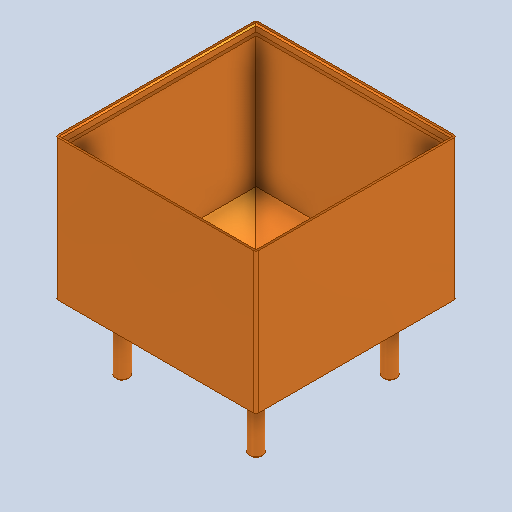
# Autodesk Inventor part: coffe container
Saved by Autodesk Inventor 2023 (Build 270158000, 158)
## iProperties
Created: 2022-11-26
Part Number: coffe container
Material: Gold
Document SubType Name: Modeling
Designer: abdul
Density: 19.3 g/cm^3
Appearance: Metal 1600F Hot
Author: abdul
Autodesk Inventor part; units mm, degrees
ref_plane "YZ Plane" through (0, 0, 0) normal (1, 0, 0) x (0, 1, 0)
ref_plane "XZ Plane" through (0, 0, 0) normal (0, 1, 0) x (-1, 0, 0)
ref_plane "XY Plane" through (0, 0, 0) normal (0, 0, 1) x (1, 0, 0)
sketch "Sketch1" plane through (0, 0, 0) normal (0, 1, 0) x (-1, 0, 0)
  line L0 (75, 75) -> (-75, 75)
  line L1 (-75, 75) -> (-75, -75)
  line L2 (-75, -75) -> (75, -75)
  line L3 (75, -75) -> (75, 75)
  point P0 (0, 0)
  dimension "d0" = 150
  dimension "d1" = 150
  dimension "d6" = 75
  dimension "d7" = 75
  constraints: 8 end point, 2 parallel, 1 horizontal, 1 perpendicular
  measures "d0" distance of L2.end L1.end
  measures "d1" distance of L1.end L0.end
  measures "d6" distance from line of L0 point (0, 0)
  measures "d7" distance from line of L3 point (0, 0)
extrude "Extrusion1" add sketch "Sketch1" along normal blind 100
sketch "Sketch2" plane through (0, 100, 0) normal (0, 1, 0) x (1, 0, 0)
  line L0 (-70, -70) -> (70, -70)
  line L1 (70, -70) -> (70, 70)
  line L2 (70, 70) -> (-70, 70)
  line L3 (-70, 70) -> (-70, -70)
  line L4 (75, 75) -> (-75, 75) projected
  line L5 (-75, -75) -> (75, -75) projected
  line L6 (-75, 75) -> (-75, -75) projected
  line L7 (75, -75) -> (75, 75) projected
  point P0 (0, 0)
  dimension "d8" = 140
  dimension "d9" = 140
  dimension "d10" = 5
  dimension "d11" = 5
  constraints: 8 end point, 6 parallel, 1 horizontal, 1 perpendicular
  measures "d8" distance of L2.end L1.end
  measures "d9" distance of L1.end L0.end
  measures "d10" distance between parallel lines of L5 L0
  measures "d11" distance between parallel lines of L6 L3
extrude "Extrusion2" cut sketch "Sketch2" against normal blind 90 contours L3 L2 L1 L0
ref_plane "Work Plane1" through (0, -50, 0) normal (0, -1, 0) x (1, 0, 0)
sketch "Sketch3" plane through (0, -50, 0) normal (0, -1, 0) x (1, 0, 0)
  circle A0 centre (0, 0) radius 15
  dimension "d15" = 30
  constraints: 1 centre point, 1 coincident
  measures "d15" diameter of A0
loft "Loft1" add profiles "Sketch3" section 2 edges at (75, 0, 0) (0, 0, 75) (-75, 0, 0) (0, 0, -75)
shell "Shell2" thickness 5 removed faces 1 at (-23.3333, 10, -23.3333)
sketch "Sketch6" plane through (0, -45, -11.4439) normal (0, 1, 0) x (0.7503372, 0, 0.6610553)
  point P0 (7.565, -8.5868)
  point P1 (7.565, -8.5868)
  constraints: 1 coincident
hole "Hole1" at (0, -45, 0) direction (0, -1, 0) diameter 50 end through all
sketch "Sketch8" plane through (0, 100, 0) normal (0, 1, 0) x (1, 0, 0)
  line L0 (-75, -75) -> (75, -75) projected
  line L1 (75, -75) -> (75, 75) projected
  line L2 (-75, -75) -> (75, -75)
  line L3 (75, -75) -> (75, 75)
  line L4 (75, 75) -> (-75, 75)
  line L5 (-75, 75) -> (-75, -75)
  point P0 (0, 0)
  constraints: 8 end point, 2 parallel, 1 horizontal, 1 perpendicular
extrude "Extrusion3" add sketch "Sketch8" along normal blind 5
sketch "Sketch9" plane through (0, 105, 0) normal (0, 1, 0) x (1, 0, 0)
  line L0 (-17.0459, -17.0459) -> (-75, -75) projected
  line L1 (17.0459, 17.0459) -> (75, 75) projected
  line L2 (-72.5, -72.5) -> (72.5, -72.5)
  line L3 (72.5, -72.5) -> (72.5, 72.5)
  line L4 (72.5, 72.5) -> (-72.5, 72.5)
  line L5 (-72.5, 72.5) -> (-72.5, -72.5)
  line L6 (75, 75) -> (-75, 75) projected
  line L7 (-75, 75) -> (-75, -75) projected
  point P0 (0, 0)
  dimension "d31" = 2.5
  dimension "d32" = 2.5
  constraints: 8 end point, 2 parallel, 2 point on line, 1 horizontal, 1 perpendicular
  measures "d31" distance between parallel lines of L6 L4
  measures "d32" distance between parallel lines of L7 L5
extrude "Extrusion4" cut sketch "Sketch9" against normal blind 5 contours L5 L4 L3 L2
chamfer "Chamfer1" distance 1 angle 45 4 edges at (-72.5, 105, 0) (0, 105, -72.5) (72.5, 105, 0) (0, 105, 72.5)
sketch "Sketch10" plane through (0, -50, 0) normal (0, -1, 0) x (1, 0, 0)
  line L0 (-17.0459, 17.0459) -> (-75, 75) projected
  circle A0 centre (-50, 50) radius 5
  line L1 (-17.0459, -17.0459) -> (-75, -75) projected
  circle A1 centre (-50, -50) radius 5
  line L2 (17.0459, -17.0459) -> (75, -75) projected
  circle A2 centre (50, -50) radius 5
  line L3 (17.0459, 17.0459) -> (75, 75) projected
  circle A3 centre (50, 50) radius 5
  point P0 (0, 0)
  dimension "d38" = 10
  dimension "d39" = 50
  dimension "d40" = 10
  dimension "d41" = 10
  dimension "d42" = 10
  constraints: 4 centre point, 4 point on line, 2 horizontal alignment, 2 vertical alignment
  measures "d38" diameter of A0
  measures "d39" horizontal distance of A0.centre point (0, 0)
  measures "d40" diameter of A1
  measures "d41" diameter of A2
  measures "d42" diameter of A3
extrude "Extrusion5" add sketch "Sketch10" against normal through all
chamfer "Chamfer2" distance 1 angle 45 4 edges at (45, -50, -50) (45, -50, 50) (-55, -50, 50) (-55, -50, -50)
fillet "Fillet1" radius 2 4 edges at (75, 52.5, -75) (-75, 52.5, -75) (-75, 52.5, 75) (75, 52.5, 75)
body "Solid1"
